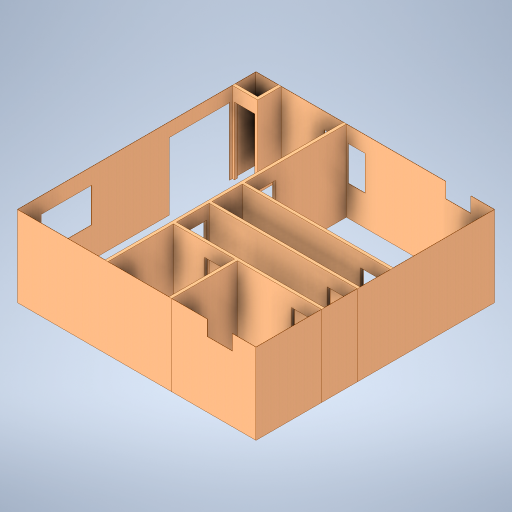
# Autodesk Inventor part: Walls--Interior--Basement
Saved by Autodesk Inventor 2024 (Build 280153000, 153)
## iProperties
Created: 2023-05-13
Part Number: Walls--Interior--Basement
Material: Generic
Document SubType Name: Modeling
Designer: Tom
Density: 1 g/cm^3
Appearance: Cherry - Natural Low Gloss
Author: Tom
Autodesk Inventor part; units mm, degrees
ref_plane "YZ Plane" through (0, 0, 0) normal (1, 0, 0) x (0, 1, 0)
ref_plane "XZ Plane" through (0, 0, 0) normal (0, 1, 0) x (-1, 0, 0)
ref_plane "XY Plane" through (0, 0, 0) normal (0, 0, 1) x (1, 0, 0)
sketch "Sketch1" plane through (0, 0, 0) normal (0, 1, 0) x (-1, 0, 0)
  line L0 (-869.95, -546.1) -> (-869.95, -457.2)
  line L1 (-869.95, 457.2) -> (-869.95, 546.1)
  line L2 (-869.95, -622.3) -> (-869.95, 622.3)
  line L3 (-958.85, 622.3) -> (-958.85, -622.3)
  line L4 (-958.85, -508) -> (-958.85, -381)
  line L5 (-869.95, -1460.5) -> (-869.95, -3600.45)
  line L6 (-958.85, -3600.45) -> (-958.85, -1460.5)
  line L7 (-3606.8, -3606.8) -> (-3606.8, 3606.8)
  line L8 (-869.95, 1460.5) -> (-869.95, 3600.45)
  line L9 (-869.95, 3606.8) -> (-958.85, 3606.8)
  line L10 (-958.85, 1460.5) -> (-869.95, 1460.5)
  line L11 (-958.85, 3600.45) -> (-958.85, 1460.5)
  line L12 (-3606.8, 3606.8) -> (3606.8, 3606.8)
  line L13 (2698.75, -457.2) -> (-869.95, -457.2)
  line L14 (-869.95, -546.1) -> (2698.75, -546.1)
  line L15 (2698.75, -546.1) -> (2698.75, -457.2)
  line L16 (3606.8, 3606.8) -> (3606.8, -3606.8)
  line L17 (2698.75, 457.2) -> (-869.95, 457.2)
  line L18 (-869.95, 546.1) -> (2698.75, 546.1)
  line L19 (2698.75, 546.1) -> (2698.75, 457.2)
  line L20 (3606.8, -3606.8) -> (-3606.8, -3606.8)
  line L21 (-869.95, -1625.6) -> (-869.95, -1536.7)
  line L22 (2698.75, -1536.7) -> (2698.75, -1625.6)
  line L23 (69.85, -1625.6) -> (-869.95, -1625.6)
  line L24 (-869.95, -1536.7) -> (69.85, -1536.7)
  line L25 (69.85, -1536.7) -> (69.85, -1625.6)
  line L26 (908.05, -1536.7) -> (908.05, -1625.6)
  line L27 (971.55, -1625.6) -> (1060.45, -1625.6)
  line L28 (908.05, -1536.7) -> (2698.75, -1536.7)
  line L29 (2698.75, -1625.6) -> (908.05, -1625.6)
  line L30 (971.55, -3600.45) -> (971.55, -1625.6)
  line L31 (1060.45, -1625.6) -> (1060.45, -3600.45)
  line L32 (-3600.45, -3600.45) -> (3600.45, -3600.45)
  line L33 (3600.45, -3600.45) -> (3600.45, 3600.45)
  line L34 (3600.45, 3600.45) -> (-3600.45, 3600.45)
  line L35 (-3600.45, 3600.45) -> (-3600.45, -3600.45)
  line L36 (-2927.35, 2978.15) -> (-2927.35, 2889.25)
  line L37 (-3600.45, 2889.25) -> (-3600.45, 2978.15)
  line L38 (-2838.45, 2889.25) -> (-2838.45, 3600.45)
  line L39 (-2838.45, 3600.45) -> (-2927.35, 3600.45)
  line L40 (-2927.35, 3600.45) -> (-2927.35, 2889.25)
  line L41 (971.55, -3600.45) -> (1060.45, -3600.45)
  line L42 (-869.95, -3600.45) -> (-958.85, -3600.45)
  line L43 (-3536.95, 2889.25) -> (-3536.95, 2978.15)
  line L44 (-3536.95, 2889.25) -> (-3600.45, 2889.25)
  line L45 (-3600.45, 2978.15) -> (-3536.95, 2978.15)
  line L46 (-2927.35, 2889.25) -> (-2838.45, 2889.25)
  line L47 (-958.85, -1460.5) -> (-869.95, -1460.5)
  line L48 (-958.85, -622.3) -> (-869.95, -622.3)
  line L49 (3600.45, -1536.7) -> (3536.95, -1536.7)
  line L50 (3536.95, -1536.7) -> (3536.95, -1625.6)
  line L51 (3536.95, -1625.6) -> (3600.45, -1625.6)
  line L52 (3600.45, -1625.6) -> (3600.45, -1536.7)
  line L53 (3600.45, -546.1) -> (3536.95, -546.1)
  line L54 (3536.95, -546.1) -> (3536.95, -457.2)
  line L55 (3536.95, -457.2) -> (3600.45, -457.2)
  line L56 (3600.45, -457.2) -> (3600.45, -546.1)
  line L57 (-958.85, 622.3) -> (-869.95, 622.3)
  line L58 (3600.45, 457.2) -> (3536.95, 457.2)
  line L59 (3536.95, 457.2) -> (3536.95, 546.1)
  line L60 (3536.95, 546.1) -> (3600.45, 546.1)
  line L61 (3600.45, 546.1) -> (3600.45, 457.2)
  point P0 (-889, -3606.8)
  point P1 (-869.95, -1625.6)
  point P2 (723.9, -3606.8)
  point P3 (-800.1, -546.1)
  point P4 (-869.95, 457.2)
  point P5 (0, 0)
  point P6 (-2927.35, 3600.45)
  point P7 (-2838.45, 3600.45)
  point P8 (1060.45, -3600.45)
  point P9 (971.55, -3600.45)
  point P10 (-869.95, -3600.45)
  point P11 (-958.85, -3600.45)
  point P12 (-869.95, -546.1)
  point P13 (3600.45, -1625.6)
  dimension "d1" = 914.4
  dimension "d7" = 1841.5
  dimension "d8" = 838.2
  dimension "d16" = 7213.6
  dimension "d17" = 7213.6
  dimension "d22" = 457.2
  dimension "d32" = 3606.8
  dimension "d33" = 6.35
  dimension "d36" = 3606.8
  dimension "d37" = 88.9
  dimension "d38" = 3568.7
  dimension "d86" = 63.5
  dimension "d87" = 711.2
  dimension "d92" = 609.6
  dimension "d106" = 76.2
  dimension "d107" = 76.2
  dimension "d110" = 838.2
  dimension "d111" = 76.2
  dimension "d112" = 838.2
  dimension "d113" = 63.5
  dimension "d121" = 838.2
  dimension "d123" = 63.5
  constraints: 124 end point, 24 collinear, 19 perpendicular, 11 point on line, 10 horizontal, 10 parallel, 9 equal length, 3 other
  measures "d1" distance between parallel lines of L17 L13
  measures "d7" distance between parallel lines of L5 L30
  measures "d8" distance between parallel lines of L26 L25
  measures "d16" distance of L20.start L20.end
  measures "d17" distance of L20.end L7.end
  measures "d22" distance from line of point (0, 0) L17
  measures "d32" distance from line of point (0, 0) L12
  measures "d33" distance between parallel lines of L12 L34
  measures "d36" distance from line of L16 point (0, 0)
  measures "d37" distance between parallel lines of L18 L17
  measures "d38" distance of L0.start L14.end
  measures "d86" distance between parallel lines of L35 L43
  measures "d87" distance of L39.end L36.end
  measures "d92" distance between parallel lines of L40 L43
  measures "d106" distance between parallel lines of L47 L24
  measures "d107" distance between parallel lines of L48 L14
  measures "d110" distance between parallel lines of L47 L48
  measures "d111" distance between parallel lines of L18 L57
  measures "d112" distance between parallel lines of L10 L57
  measures "d113" distance between parallel lines of L52 L50
  measures "d121" distance between parallel lines of L22 L50
  measures "d123" distance between parallel lines of L26 L30
extrude "Extrusion1" add sketch "Sketch1" along normal blind 2438.4 contours L2 L48 L3 L57 L1 L0 | L0 L13 L15 L14 | L1 L18 L19 L17 | L5 L32 L6 L47 | L24 L25 L23 L5 | L30 L27 L31 L32 | L35 L45 L43 L44 | L29 L26 L28 L22 L27 | L51 L50 L49 L33 | L34 L38 L46 L36 L40 | L53 L54 L55 L33 | L34 L8 L10 L11 | L58 L59 L60 L33 | L7 L12 L9 L16 L20
sketch "Sketch2" plane through (3606.8, 0, -3606.8) normal (0, 0, -1) x (-1, 0, 0)
  line L0 (7213.6, 2438.4) -> (0, 2438.4) projected
  line L1 (6502.4, 2438.4) -> (5740.4, 2438.4)
  line L2 (5740.4, 2438.4) -> (5740.4, 1981.2)
  line L3 (5740.4, 1981.2) -> (6502.4, 1981.2)
  line L4 (6502.4, 1981.2) -> (6502.4, 2438.4)
  line L5 (7213.6, 0) -> (7213.6, 2438.4) projected
  point P0 (3606.8, 0)
  point P1 (5740.4, 2438.4)
  dimension "d41" = 711.2
  dimension "d42" = 762
  dimension "d43" = 457.2
  constraints: 8 end point, 2 parallel, 1 horizontal, 1 perpendicular, 1 point on line
  measures "d41" distance between parallel lines of L5 L4
  measures "d42" distance of L2.end L3.end
  measures "d43" distance of L1.end L2.end
extrude "Extrusion2" cut sketch "Sketch2" against normal up to surface (6.35 mm away)
sketch "Sketch3" plane through (869.95, 0, 3600.45) normal (0, 0, -1) x (-1, 0, 0)
  line L0 (63.5, 1955.8) -> (571.5, 1955.8)
  line L1 (571.5, 1955.8) -> (571.5, 914.4)
  line L2 (571.5, 914.4) -> (63.5, 914.4)
  line L3 (63.5, 914.4) -> (63.5, 1955.8)
  line L4 (0, 0) -> (-88.9, 0) projected
  line L5 (0, 0) -> (0, 2438.4) projected
  point P0 (4470.4, 0)
  dimension "d48" = 1041.4
  dimension "d49" = 508
  dimension "d50" = 914.4
  dimension "d51" = 63.5
  constraints: 8 end point, 2 parallel, 1 horizontal, 1 perpendicular
  measures "d48" distance of L0.end L1.end
  measures "d49" distance of L0.start L0.end
  measures "d50" distance between parallel lines of L4 L2
  measures "d51" distance between parallel lines of L5 L3
extrude "Extrusion3" cut sketch "Sketch3" against normal up to surface (6.35 mm away)
sketch "Sketch4" plane through (869.95, 0, 3600.45) normal (0, 0, -1) x (-1, 0, 0)
  line L0 (3765.55, 2438.4) -> (3003.55, 2438.4)
  line L1 (3003.55, 2438.4) -> (3003.55, 1981.2)
  line L2 (3003.55, 1981.2) -> (3765.55, 1981.2)
  line L3 (3765.55, 1981.2) -> (3765.55, 2438.4)
  line L4 (4470.4, 0) -> (4470.4, 2438.4) projected
  line L5 (0, 2438.4) -> (-88.9, 2438.4) projected
  point P0 (869.95, 0)
  point P1 (4476.75, 2438.4)
  dimension "d55" = 457.2
  dimension "d56" = 762
  dimension "d85" = 711.2
  constraints: 8 end point, 2 parallel, 1 collinear, 1 horizontal, 1 perpendicular
  measures "d55" distance of L0.end L1.end
  measures "d56" distance of L1.end L2.end
  measures "d85" distance from line of point (4476.75, 2438.4) L3
extrude "Extrusion4" cut sketch "Sketch4" against normal up to surface (6.35 mm away)
sketch "Sketch5" plane through (2838.45, 0, 3600.45) normal (0, 0, -1) x (-1, 0, 0)
  line L0 (1816.1, 1955.8) -> (1308.1, 1955.8)
  line L1 (1308.1, 1955.8) -> (1308.1, 914.4)
  line L2 (1308.1, 914.4) -> (1816.1, 914.4)
  line L3 (1816.1, 914.4) -> (1816.1, 1955.8)
  line L4 (1879.6, 0) -> (1879.6, 2438.4) projected
  line L5 (0, 0) -> (1879.6, 0) projected
  point P0 (2838.45, 0)
  dimension "d60" = 63.5
  dimension "d61" = 914.4
  dimension "d62" = 508
  dimension "d63" = 1041.4
  constraints: 8 end point, 2 parallel, 1 horizontal, 1 perpendicular
  measures "d60" distance between parallel lines of L4 L3
  measures "d61" distance between parallel lines of L5 L2
  measures "d62" distance of L0.start L0.end
  measures "d63" distance of L0.end L1.end
extrude "Extrusion5" cut sketch "Sketch5" against normal up to surface (6.35 mm away)
sketch "Sketch6" plane through (3600.45, 0, -3600.45) normal (-1, 0, 0) x (0, 0, 1)
  line L0 (6578.6, 0) -> (6489.7, 0) projected
  line L1 (6578.6, 0) -> (4578.35, 0)
  line L2 (4578.35, 0) -> (4578.35, 2032)
  line L3 (4578.35, 2032) -> (6407.15, 2032)
  line L4 (6489.7, 0) -> (6489.7, 2438.4) projected
  line L5 (6407.15, 2032) -> (6407.15, 0)
  point P0 (3600.45, 0)
  point P1 (0, 0)
  point P2 (4572, 0)
  point P3 (7200.9, 0)
  dimension "d68" = 1828.8
  dimension "d69" = 2032
  dimension "d122" = 82.55
  constraints: 9 end point, 2 perpendicular, 1 horizontal, 1 parallel, 1 point on line
  measures "d68" distance of L2.end L3.end
  measures "d69" distance of L1.end L2.end
  measures "d122" distance between parallel lines of L5 L4
extrude "Extrusion6" cut sketch "Sketch6" against normal up to surface (6.35 mm away)
sketch "Sketch7" plane through (3600.45, 0, 2889.25) normal (-1, 0, 0) x (0, 0, 1)
  line L0 (-5784.85, 1955.8) -> (-4260.85, 1955.8)
  line L1 (-4260.85, 1955.8) -> (-4260.85, 914.4)
  line L2 (-4260.85, 914.4) -> (-5784.85, 914.4)
  line L3 (-5784.85, 914.4) -> (-5784.85, 1955.8)
  line L4 (88.9, 0) -> (0, 0) projected
  line L5 (-6489.7, 0) -> (-6489.7, 2438.4) projected
  point P0 (-2889.25, 0)
  point P1 (-1911.35, 0)
  dimension "d74" = 1524
  dimension "d75" = 914.4
  dimension "d76" = 704.85
  constraints: 8 end point, 2 parallel, 1 horizontal, 1 perpendicular
  measures "d74" distance of L0.start L0.end
  measures "d75" distance between parallel lines of L4 L2
  measures "d76" distance between parallel lines of L5 L3
extrude "Extrusion7" cut sketch "Sketch7" against normal up to surface (6.35 mm away)
sketch "Sketch8" plane through (-69.85, 0, -1625.6) normal (-1, 0, 0) x (0, 0, 1)
  line L0 (0, 2438.4) -> (88.9, 2438.4) projected
  line L1 (88.9, 0) -> (88.9, 2438.4) projected
  line L2 (0, 2438.4) -> (88.9, 2438.4)
  line L3 (88.9, 2438.4) -> (88.9, 2032)
  line L4 (88.9, 2032) -> (0, 2032)
  line L5 (0, 2032) -> (0, 2438.4)
  point P0 (1625.6, 0)
  dimension "d79" = 406.4
  constraints: 8 end point, 2 parallel, 1 horizontal, 1 perpendicular, 1 point on line
  measures "d79" distance between parallel lines of L0 L4
extrude "Extrusion8" add sketch "Sketch8" along normal up to surface (838.2 mm away)
sketch "Sketch9" plane through (-2698.75, 0, -1625.6) normal (-1, 0, 0) x (0, 0, 1)
  line L0 (0, 0) -> (0, 2438.4) projected
  line L1 (88.9, 0) -> (88.9, 2438.4) projected
  line L2 (0, 2032) -> (88.9, 2032)
  line L3 (88.9, 2032) -> (88.9, 2438.4)
  line L4 (88.9, 2438.4) -> (0, 2438.4)
  line L5 (0, 2438.4) -> (0, 2032)
  point P0 (1625.6, 0)
  point P1 (88.9, 2032)
  point P2 (44.45, 2032)
  dimension "d84" = 406.4
  constraints: 8 end point, 2 parallel, 1 horizontal, 1 midpoint, 1 perpendicular, 1 point on line
  measures "d84" distance from line of L4 point (44.45, 2032)
extrude "Extrusion9" add sketch "Sketch9" along normal up to surface (901.7 mm away)
sketch "Sketch10" plane through (3536.95, 0, 2889.25) normal (-1, 0, 0) x (0, 0, 1)
  line L0 (88.9, 0) -> (88.9, 2438.4) projected
  line L1 (0, 0) -> (0, 2438.4) projected
  line L2 (88.9, 2032) -> (0, 2032)
  line L3 (0, 2032) -> (0, 2438.4)
  line L4 (0, 2438.4) -> (88.9, 2438.4)
  line L5 (88.9, 2438.4) -> (88.9, 2032)
  point P0 (-2889.25, 0)
  point P1 (0, 2032)
  dimension "d94" = 406.4
  constraints: 8 end point, 2 parallel, 1 horizontal, 1 perpendicular, 1 point on line
  measures "d94" distance between parallel lines of L4 L2
extrude "Extrusion10" add sketch "Sketch10" along normal up to surface (609.6 mm away)
sketch "Sketch11" plane through (-2698.75, 0, 457.2) normal (-1, 0, 0) x (0, 0, 1)
  line L0 (88.9, 0) -> (88.9, 2438.4) projected
  line L1 (0, 0) -> (0, 2438.4) projected
  line L2 (88.9, 2032) -> (0, 2032)
  line L3 (0, 2032) -> (0, 2438.4)
  line L4 (0, 2438.4) -> (88.9, 2438.4)
  line L5 (88.9, 2438.4) -> (88.9, 2032)
  point P0 (-457.2, 0)
  point P1 (0, 2032)
  dimension "d97" = 406.4
  constraints: 8 end point, 2 parallel, 1 horizontal, 1 perpendicular, 1 point on line
  measures "d97" distance between parallel lines of L4 L2
extrude "Extrusion11" add sketch "Sketch11" along normal up to surface (901.7 mm away)
sketch "Sketch12" plane through (-2698.75, 0, -546.1) normal (-1, 0, 0) x (0, 0, 1)
  line L0 (88.9, 0) -> (88.9, 2438.4) projected
  line L1 (0, 2438.4) -> (88.9, 2438.4) projected
  line L2 (88.9, 2032) -> (0, 2032)
  line L3 (0, 2032) -> (0, 2438.4)
  line L4 (0, 2438.4) -> (88.9, 2438.4)
  line L5 (88.9, 2438.4) -> (88.9, 2032)
  point P0 (546.1, 0)
  dimension "d100" = 406.4
  constraints: 8 end point, 2 parallel, 1 horizontal, 1 perpendicular, 1 point on line
  measures "d100" distance between parallel lines of L1 L2
extrude "Extrusion12" add sketch "Sketch12" along normal up to surface (901.7 mm away)
sketch "Sketch15" plane through (958.85, 0, 1460.5) normal (0, 0, -1) x (-1, 0, 0)
  line L0 (88.9, 0) -> (88.9, 2438.4) projected
  line L1 (0, 2438.4) -> (88.9, 2438.4) projected
  line L2 (88.9, 2032) -> (0, 2032)
  line L3 (0, 2032) -> (0, 2438.4)
  line L4 (0, 2438.4) -> (88.9, 2438.4)
  line L5 (88.9, 2438.4) -> (88.9, 2032)
  point P0 (958.85, 0)
  dimension "d115" = 406.4
  constraints: 8 end point, 2 parallel, 1 horizontal, 1 perpendicular, 1 point on line
  measures "d115" distance between parallel lines of L1 L2
extrude "Extrusion14" add sketch "Sketch15" along normal up to surface (838.2 mm away)
sketch "Sketch16" plane through (869.95, 0, -1460.5) normal (0, 0, 1) x (1, 0, 0)
  line L0 (0, 0) -> (0, 2438.4) projected
  line L1 (88.9, 0) -> (88.9, 2438.4) projected
  line L2 (0, 2438.4) -> (88.9, 2438.4)
  line L3 (88.9, 2438.4) -> (88.9, 2032)
  line L4 (88.9, 2032) -> (0, 2032)
  line L5 (0, 2032) -> (0, 2438.4)
  point P0 (-869.95, 0)
  point P1 (88.9, 2438.4)
  point P2 (0, 2032)
  dimension "d118" = 406.4
  constraints: 8 end point, 2 parallel, 1 horizontal, 1 perpendicular, 1 point on line
  measures "d118" distance between parallel lines of L2 L4
extrude "Extrusion15" add sketch "Sketch16" along normal up to surface (838.2 mm away)
body "Solid1"
